Autodesk Fusion 360 part; units mm, degrees
(part 2 of 3)
  line L880 (190.4485, 318.4129) -> (189.5942, 317.9397)
  line L881 (195.3697, 320.9495) -> (194.2984, 320.4242)
  line L882 (211.6798, 327.3307) -> (210.0741, 326.8246)
  line L883 (186.8285, 281.1395) -> (187.261, 279.1724)
  line L884 (184.9285, 291.0204) -> (185.2733, 289.0389)
  line L885 (187.2886, 316.6135) -> (186.3635, 316.0568)
  line L886 (182.4919, 313.4456) -> (182.399, 313.3626)
  line L887 (185.6357, 287.0598) -> (186.0157, 285.0834)
  line L888 (213.3309, 327.826) -> (211.6798, 327.3307)
  line L889 (243.1905, 182.1136) -> (244.2111, 181.3414)
  line L890 (211.4232, 217.808) -> (212.1963, 216.5757)
  line L891 (204.1026, 324.7205) -> (202.7219, 324.1817)
  line L892 (214.5928, 212.9181) -> (215.4171, 211.7129)
  line L893 (186.0157, 285.0834) -> (186.4134, 283.1099)
  line L894 (196.4887, 248.3332) -> (197.2058, 246.4567)
  line L895 (192.2867, 319.3977) -> (191.346, 318.8994)
  line L896 (182.3588, 313.0956) -> (182.3533, 312.8495)
  line L897 (221.5355, 203.5012) -> (222.4584, 202.3634)
  line L898 (228.1911, 331.2302) -> (227.1757, 331.054)
  line L899 (182.734, 313.6258) -> (182.4919, 313.4456)
  line L900 (229.2183, 331.4005) -> (228.1911, 331.2302)
  line L901 (210.0741, 326.8246) -> (208.5136, 326.3091)
  line L902 (198.8469, 322.5569) -> (197.6438, 322.0173)
  line L903 (186.4134, 283.1099) -> (186.8285, 281.1395)
  line L904 (182.3533, 312.8495) -> (182.3576, 312.5288)
  line L905 (205.528, 325.2557) -> (204.1026, 324.7205)
  line L906 (190.7699, 265.5148) -> (191.339, 263.5824)
  line L907 (185.4486, 315.4831) -> (184.5455, 314.8912)
  line L908 (191.346, 318.8994) -> (190.4485, 318.4129)
  line L909 (182.3964, 311.6644) -> (182.4765, 310.5043)
  line L910 (230.2661, 193.6329) -> (231.294, 192.5922)
  line L911 (241.0426, 183.8051) -> (242.1796, 182.8983)
  line L912 (187.261, 279.1724) -> (187.7108, 277.2089)
  line L913 (206.4443, 226.1875) -> (206.7996, 225.5399)
  line L914 (183.2362, 302.9484) -> (183.4731, 300.9569)
  line L915 (194.4344, 254.0045) -> (195.1029, 252.1073)
  line L916 (212.1963, 216.5757) -> (212.9823, 215.3497)
  line L917 (222.4584, 202.3634) -> (223.3933, 201.2354)
  line L918 (184.2925, 294.9899) -> (184.6016, 293.0042)
  line L919 (226.1718, 330.8721) -> (224.199, 330.492)
  line L920 (213.7812, 214.1305) -> (214.5928, 212.9181)
  line L921 (229.2496, 194.6856) -> (230.2661, 193.6329)
  line L922 (231.3075, 331.7228) -> (230.2571, 331.5647)
  line L923 (194.2984, 320.4242) -> (193.2708, 319.9065)
  line L924 (208.9796, 221.8036) -> (209.7164, 220.5848)
  line L925 (200.196, 239.0794) -> (200.5746, 238.1864)
  line L926 (216.254, 210.5152) -> (217.1034, 209.3252)
  line L927 (198.1538, 320.0225) -> (199.198, 320.4971)
  line L928 (237.6951, 186.6124) -> (238.8002, 185.6625)
  line L929 (196.3039, 254.6319) -> (195.6779, 256.4565)
  line L930 (239.9161, 184.7266) -> (241.0426, 183.8051)
  line L931 (186.1932, 295.8614) -> (185.9184, 297.7719)
  line L932 (184.8426, 312.7237) -> (185.3358, 313.0673)
  line L933 (192.5275, 259.7337) -> (193.1466, 257.8179)
  line L934 (191.2359, 271.2561) -> (190.7519, 273.1282)
  line L935 (246.2732, 179.825) -> (248.1998, 178.4241)
  line L936 (191.7358, 269.3885) -> (191.2359, 271.2561)
  line L937 (189.3954, 278.7688) -> (188.9752, 280.6564)
  line L938 (189.8316, 276.8847) -> (189.3954, 278.7688)
  line L939 (189.6821, 269.3948) -> (190.2176, 267.4524)
  line L940 (184.4092, 311.5322) -> (184.3858, 311.947)
  line L941 (198.2755, 249.1965) -> (197.6027, 251.0016)
  line L942 (215.4171, 211.7129) -> (216.254, 210.5152)
  line L943 (195.1029, 252.1073) -> (195.7877, 250.2168)
  line L944 (195.0675, 258.2873) -> (194.4728, 260.124)
  line L945 (244.2111, 181.3414) -> (245.2393, 180.5793)
  line L946 (224.3401, 200.1173) -> (225.2987, 199.0094)
  line L947 (185.1917, 303.5112) -> (184.9822, 305.4263)
  line L948 (188.6623, 273.2934) -> (189.1637, 271.3419)
  line L949 (197.9391, 244.5874) -> (198.6883, 242.7258)
  line L950 (225.2987, 199.0094) -> (226.269, 197.912)
  line L951 (228.2445, 195.7498) -> (229.2496, 194.6856)
  line L952 (207.737, 223.9002) -> (208.3199, 222.9089)
  line L953 (232.3331, 191.5636) -> (233.3834, 190.5474)
  line L954 (195.7877, 250.2168) -> (196.4887, 248.3332)
  line L955 (189.1637, 271.3419) -> (189.6821, 269.3948)
  line L956 (233.3834, 190.5474) -> (234.4449, 189.5439)
  line L957 (218.8395, 206.9696) -> (219.726, 205.8045)
  line L958 (193.7823, 255.9081) -> (194.4344, 254.0045)
  line L959 (217.1034, 209.3252) -> (217.9652, 208.1433)
  line L960 (236.6008, 187.5761) -> (237.6951, 186.6124)
  line L961 (200.9684, 237.3) -> (206.4443, 226.1875)
  line L962 (188.178, 275.2492) -> (188.6623, 273.2934)
  line L963 (196.9455, 252.8135) -> (196.3039, 254.6319)
  line L964 (192.2516, 267.5255) -> (191.7358, 269.3885)
  line L965 (223.3933, 201.2354) -> (224.3401, 200.1173)
  line L966 (191.339, 263.5824) -> (191.9249, 261.6553)
  line L967 (200.5746, 238.1864) -> (200.9684, 237.3)
  line L968 (199.198, 320.4971) -> (200.2826, 320.9764)
  line L969 (188.1829, 284.4416) -> (187.8109, 286.3388)
  line L970 (187.455, 288.2387) -> (187.1153, 290.1411)
  line L971 (193.3307, 263.8142) -> (192.7833, 265.6673)
  line L972 (184.3824, 312.2188) -> (184.3884, 312.3009)
  line L973 (190.2837, 275.0044) -> (189.8316, 276.8847)
  line L974 (192.7833, 265.6673) -> (192.2516, 267.5255)
  line L975 (198.6883, 242.7258) -> (199.4535, 240.8719)
  line L976 (209.7164, 220.5848) -> (210.5308, 219.2528)
  line L977 (206.7996, 225.5399) -> (207.2303, 224.7774)
  line L978 (219.726, 205.8045) -> (220.6247, 204.6483)
  line L979 (210.5308, 219.2528) -> (211.4232, 217.808)
  line L980 (212.9823, 215.3497) -> (213.7812, 214.1305)
  line L981 (208.3199, 222.9089) -> (208.9796, 221.8036)
  line L982 (199.4535, 240.8719) -> (200.196, 239.0794)
  line L983 (207.2303, 224.7774) -> (207.737, 223.9002)
  line L984 (235.5173, 188.5534) -> (236.6008, 187.5761)
  line L985 (231.294, 192.5922) -> (232.3331, 191.5636)
  line L986 (190.2176, 267.4524) -> (190.7699, 265.5148)
  line L987 (191.9249, 261.6553) -> (192.5275, 259.7337)
  line L988 (227.251, 196.8254) -> (228.2445, 195.7498)
  line L989 (238.8002, 185.6625) -> (239.9161, 184.7266)
  line L990 (220.6247, 204.6483) -> (221.5355, 203.5012)
  line L991 (187.8109, 286.3388) -> (187.455, 288.2387)
  line L992 (245.2393, 180.5793) -> (246.2732, 179.825)
  line L993 (294.5657, 322.5161) -> (295.4347, 322.1728)
  line L994 (191.9665, 316.9376) -> (193.5353, 317.764)
  line L995 (278.8099, 327.5376) -> (279.9258, 327.2443)
  line L996 (186.8702, 314.0439) -> (187.9132, 314.6687)
  line L997 (184.4516, 310.9753) -> (184.4092, 311.5322)
  line L998 (238.245, 330.6174) -> (239.0438, 330.7015)
  line L999 (240.3196, 330.8043) -> (258.3534, 330.7921)
  line L1000 (261.8335, 330.4341) -> (263.5877, 330.2118)
  line L1001 (232.6443, 329.8932) -> (235.2057, 330.2411)
  line L1002 (187.1153, 290.1411) -> (186.7917, 292.0458)
  line L1003 (185.9184, 297.7719) -> (185.6598, 299.6838)
  line L1004 (184.3999, 312.3469) -> (184.4429, 312.401)
  line L1005 (187.9132, 314.6687) -> (189.1413, 315.3788)
  line L1006 (184.5888, 309.4382) -> (184.4516, 310.9753)
  line L1007 (197.15, 319.5539) -> (198.1538, 320.0225)
  line L1008 (193.8939, 261.9664) -> (193.3307, 263.8142)
  line L1009 (190.7519, 273.1282) -> (190.2837, 275.0044)
  line L1010 (184.4429, 312.401) -> (184.5309, 312.4822)
  line L1011 (184.3858, 311.947) -> (184.3824, 312.2188)
  line L1012 (248.8662, 177.9546) -> (248.9417, 177.9125)
  line L1013 (210.4325, 324.8283) -> (211.8874, 325.2931)
  line L1014 (206.3175, 323.399) -> (207.6477, 323.88)
  line L1015 (223.2492, 328.2546) -> (225.0422, 328.6208)
  line L1016 (269.5072, 329.3395) -> (270.9528, 329.1031)
  line L1017 (195.6779, 256.4565) -> (195.0675, 258.2873)
  line L1018 (188.9752, 280.6564) -> (188.571, 282.5475)
  line L1019 (195.2628, 318.6395) -> (196.1863, 319.0925)
  line L1020 (258.3534, 330.7921) -> (258.6905, 330.7668)
  line L1021 (270.9528, 329.1031) -> (272.0957, 328.9193)
  line L1022 (218.1261, 327.0605) -> (219.7913, 327.4732)
  line L1023 (194.3791, 318.1963) -> (195.2628, 318.6395)
  line L1024 (239.0438, 330.7015) -> (239.7353, 330.7641)
  line L1025 (275.5164, 328.3239) -> (276.1633, 328.1825)
  line L1026 (259.3837, 330.7039) -> (260.4318, 330.5955)
  line L1027 (283.9678, 326.1106) -> (285.7506, 325.5765)
  line L1028 (198.9639, 247.3984) -> (198.2755, 249.1965)
  line L1029 (295.4347, 322.1728) -> (296.301, 321.8224)
  line L1030 (203.7807, 322.4298) -> (205.0285, 322.9152)
  line L1031 (207.6477, 323.88) -> (209.0193, 324.3568)
  line L1032 (190.5552, 316.1702) -> (191.9665, 316.9376)
  line L1033 (184.9822, 305.4263) -> (184.7891, 307.3421)
  line L1034 (194.4728, 260.124) -> (193.8939, 261.9664)
  line L1035 (185.4176, 301.597) -> (185.1917, 303.5112)
  line L1036 (248.1998, 178.4241) -> (248.7176, 178.0543)
  line L1037 (186.4843, 293.9527) -> (186.1932, 295.8614)
  line L1038 (185.3358, 313.0673) -> (186.0113, 313.5087)
  line L1039 (197.6027, 251.0016) -> (196.9455, 252.8135)
  line L1040 (196.1863, 319.0925) -> (197.15, 319.5539)
  line L1041 (248.7176, 178.0543) -> (248.8662, 177.9546)
  line L1042 (184.3884, 312.3009) -> (184.3999, 312.3469)
  line L1043 (193.5353, 317.764) -> (194.3791, 318.1963)
  line L1044 (184.7891, 307.3421) -> (184.5888, 309.4382)
  line L1045 (188.571, 282.5475) -> (188.1829, 284.4416)
  line L1046 (272.0957, 328.9193) -> (273.2392, 328.7379)
  line L1047 (189.1413, 315.3788) -> (190.5552, 316.1702)
  line L1048 (184.5309, 312.4822) -> (184.8426, 312.7237)
  line L1049 (185.6598, 299.6838) -> (185.4176, 301.597)
  line L1050 (298.8814, 320.7283) -> (299.7349, 320.349)
  line L1051 (300.5849, 319.9624) -> (301.4312, 319.5683)
  line L1052 (211.8874, 325.2931) -> (213.384, 325.7499)
  line L1053 (186.0113, 313.5087) -> (186.8702, 314.0439)
  line L1054 (186.7917, 292.0458) -> (186.4843, 293.9527)
  line L1055 (209.0193, 324.3568) -> (210.4325, 324.8283)
  line L1056 (265.6932, 329.921) -> (268.1486, 329.554)
  line L1057 (277.8105, 327.7908) -> (278.8099, 327.5376)
  line L1058 (239.7353, 330.7641) -> (240.3196, 330.8043)
  line L1059 (202.5738, 321.944) -> (203.7807, 322.4298)
  line L1060 (260.4318, 330.5955) -> (261.8335, 330.4341)
  line L1061 (228.757, 329.298) -> (230.679, 329.6065)
  line L1062 (291.064, 323.8204) -> (292.8196, 323.182)
  line L1063 (298.0244, 321.1002) -> (298.8814, 320.7283)
  line L1064 (313.6797, 306.995) -> (313.501, 305.1643)
  line L1065 (302.2738, 319.1668) -> (303.1123, 318.7576)
  line L1066 (313.8935, 309.2436) -> (313.6797, 306.995)
  line L1067 (312.0915, 294.2029) -> (311.8012, 292.3814)
  line L1068 (273.2392, 328.7379) -> (274.3804, 328.5443)
  line L1069 (276.9282, 328.0053) -> (277.8105, 327.7908)
  line L1070 (219.7913, 327.4732) -> (221.499, 327.8716)
  line L1071 (305.6295, 265.399) -> (305.1009, 263.6307)
  line L1072 (312.4719, 313.4707) -> (313.3652, 312.9061)
  line L1073 (314.1337, 311.9322) -> (314.0498, 310.8908)
  line L1074 (313.306, 303.3344) -> (313.095, 301.5055)
  line L1075 (299.7349, 320.349) -> (300.5849, 319.9624)
  line L1076 (313.9209, 312.5379) -> (314.0694, 312.4265)
  line L1077 (201.4079, 321.4591) -> (202.5738, 321.944)
  line L1078 (301.0102, 251.3972) -> (300.3711, 249.6723)
  line L1079 (307.2409, 316.5958) -> (308.0528, 316.1398)
  line L1080 (221.499, 327.8716) -> (223.2492, 328.2546)
  line L1081 (226.8781, 328.9691) -> (228.757, 329.298)
  line L1082 (292.8196, 323.182) -> (294.5657, 322.5161)
  line L1083 (258.6905, 330.7668) -> (259.3837, 330.7039)
  line L1084 (214.9226, 326.1977) -> (216.5032, 326.6349)
  line L1085 (205.0285, 322.9152) -> (206.3175, 323.399)
  line L1086 (230.679, 329.6065) -> (232.6443, 329.8932)
  line L1087 (263.5877, 330.2118) -> (265.6932, 329.921)
  line L1088 (268.1486, 329.554) -> (269.5072, 329.3395)
  line L1089 (274.3804, 328.5443) -> (274.9492, 328.4384)
  line L1090 (308.9263, 277.8968) -> (308.4991, 276.0998)
  line L1091 (305.6029, 317.484) -> (306.4242, 317.0439)
  line L1092 (307.1295, 270.7309) -> (306.6439, 268.9492)
  line L1093 (312.6249, 297.8512) -> (312.3661, 296.0262)
  line L1094 (309.6616, 315.2036) -> (310.4583, 314.7233)
  line L1095 (311.4954, 290.5619) -> (311.1741, 288.7447)
  line L1096 (310.4854, 285.1174) -> (310.1182, 283.3078)
  line L1097 (310.1182, 283.3078) -> (309.7359, 281.501)
  line L1098 (305.1009, 263.6307) -> (304.5582, 261.8672)
  line L1099 (303.9468, 318.3408) -> (304.777, 317.9163)
  line L1100 (213.384, 325.7499) -> (214.9226, 326.1977)
  line L1101 (279.9258, 327.2443) -> (281.1578, 326.9097)
  line L1102 (308.0528, 316.1398) -> (308.8598, 315.6758)
  line L1103 (287.5283, 325.0171) -> (289.2998, 324.4319)
  line L1104 (311.8012, 292.3814) -> (311.4954, 290.5619)
  line L1105 (282.5052, 326.5322) -> (283.9678, 326.1106)
  line L1106 (314.1303, 312.3631) -> (314.1401, 312.3128)
  line L1107 (274.9492, 328.4384) -> (275.5164, 328.3239)
  line L1108 (200.2826, 320.9764) -> (201.4079, 321.4591)
  line L1109 (237.339, 330.5122) -> (238.245, 330.6174)
  line L1110 (216.5032, 326.6349) -> (218.1261, 327.0605)
  line L1111 (281.1578, 326.9097) -> (282.5052, 326.5322)
  line L1112 (285.7506, 325.5765) -> (287.5283, 325.0171)
  line L1113 (276.1633, 328.1825) -> (276.9282, 328.0053)
  line L1114 (289.2998, 324.4319) -> (291.064, 323.8204)
  line L1115 (297.1643, 321.4649) -> (298.0244, 321.1002)
  line L1116 (225.0422, 328.6208) -> (226.8781, 328.9691)
  line L1117 (235.2057, 330.2411) -> (237.339, 330.5122)
  line L1118 (296.301, 321.8224) -> (297.1643, 321.4649)
  line L1119 (306.6439, 268.9492) -> (306.1438, 267.1719)
  line L1120 (314.1401, 312.3128) -> (314.1439, 312.2242)
  line L1121 (236.8455, 190.0948) -> (235.7247, 191.1305)
  line L1122 (310.4583, 314.7233) -> (311.2496, 314.2347)
  line L1123 (308.4991, 276.0998) -> (308.0572, 274.3063)
  line L1124 (306.1438, 267.1719) -> (305.6295, 265.399)
  line L1125 (303.4307, 258.3554) -> (302.8462, 256.6074)
  line L1126 (279.9298, 210.7253) -> (278.7353, 209.0622)
  line L1127 (249.2499, 180.1523) -> (249.1978, 180.174)
  line L1128 (256.2407, 185.4395) -> (255.1379, 184.5517)
  line L1129 (313.095, 301.5055) -> (312.8679, 299.6777)
  line L1130 (296.9792, 241.1186) -> (296.282, 239.4885)
  line L1131 (288.4746, 223.9458) -> (287.906, 222.9657)
  line L1132 (313.3652, 312.9061) -> (313.9209, 312.5379)
  line L1133 (302.8462, 256.6074) -> (302.2478, 254.8649)
  line L1134 (303.1123, 318.7576) -> (303.9468, 318.3408)
  line L1135 (302.2478, 254.8649) -> (301.6358, 253.1281)
  line L1136 (295.0943, 236.8299) -> (294.6113, 235.7987)
  line L1137 (261.7197, 190.1093) -> (259.4933, 188.169)
  line L1138 (314.1109, 312.3888) -> (314.1303, 312.3631)
  line L1139 (249.3666, 180.2174) -> (249.2896, 180.1687)
  line L1140 (237.9781, 189.0732) -> (236.8455, 190.0948)
  line L1141 (265.5721, 193.6166) -> (264.9971, 193.0698)
  line L1142 (264.9971, 193.0698) -> (264.3244, 192.4454)
  line L1143 (234.6159, 192.1801) -> (233.5192, 193.2433)
  line L1144 (281.1036, 212.4027) -> (279.9298, 210.7253)
  line L1145 (288.9441, 224.778) -> (288.4746, 223.9458)
  line L1146 (309.7359, 281.501) -> (309.3385, 279.6973)
  line L1147 (301.6358, 253.1281) -> (301.0102, 251.3972)
  line L1148 (308.8598, 315.6758) -> (309.6616, 315.2036)
  line L1149 (250.627, 181.1318) -> (249.6337, 180.4076)
  line L1150 (257.334, 186.3388) -> (256.2407, 185.4395)
  line L1151 (233.5192, 193.2433) -> (232.4347, 194.3197)
  line L1152 (232.4347, 194.3197) -> (231.3627, 195.4091)
  line L1153 (313.501, 305.1643) -> (313.306, 303.3344)
  line L1154 (278.1296, 208.2367) -> (277.5179, 207.4156)
  line L1155 (307.6006, 272.5166) -> (307.1295, 270.7309)
  line L1156 (242.6238, 185.134) -> (241.4454, 186.0962)
  line L1157 (254.0255, 183.6763) -> (252.903, 182.814)
  line L1158 (245.0138, 183.2568) -> (243.8133, 184.1875)
  line L1159 (272.3827, 201.043) -> (266.0497, 194.0855)
  line L1160 (314.0498, 310.8908) -> (313.8935, 309.2436)
  line L1161 (301.4312, 319.5683) -> (302.2738, 319.1668)
  line L1162 (249.0969, 180.2383) -> (248.7472, 180.4891)
  line L1163 (314.1439, 312.2242) -> (314.1337, 311.9322)
  line L1164 (298.562, 244.9862) -> (297.7405, 242.9507)
  line L1165 (297.7405, 242.9507) -> (296.9792, 241.1186)
  line L1166 (239.1223, 188.066) -> (237.9781, 189.0732)
  line L1167 (314.0694, 312.4265) -> (314.1109, 312.3888)
  line L1168 (308.0572, 274.3063) -> (307.6006, 272.5166)
  line L1169 (311.1741, 288.7447) -> (310.8374, 286.9298)
  line L1170 (299.4401, 247.2263) -> (298.562, 244.9862)
  line L1171 (312.3661, 296.0262) -> (312.0915, 294.2029)
  line L1172 (310.8374, 286.9298) -> (310.4854, 285.1174)
  line L1173 (309.3385, 279.6973) -> (308.9263, 277.8968)
  line L1174 (304.5582, 261.8672) -> (304.0014, 260.1087)
  line L1175 (306.4242, 317.0439) -> (307.2409, 316.5958)
  line L1176 (312.8679, 299.6777) -> (312.6249, 297.8512)
  line L1177 (311.2496, 314.2347) -> (312.4719, 313.4707)
  line L1178 (300.3711, 249.6723) -> (299.4401, 247.2263)
  line L1179 (304.777, 317.9163) -> (305.6029, 317.484)
  line L1180 (295.6525, 238.0594) -> (295.0943, 236.8299)
  line L1181 (304.0014, 260.1087) -> (303.4307, 258.3554)
  line L1182 (296.282, 239.4885) -> (295.6525, 238.0594)
  line L1183 (274.3625, 203.3875) -> (273.7102, 202.5994)
  line L1184 (249.2896, 180.1687) -> (249.2499, 180.1523)
  line L1185 (287.2355, 221.8397) -> (286.4604, 220.5699)
  line L1186 (243.8133, 184.1875) -> (242.6238, 185.134)
  line L1187 (248.7472, 180.4891) -> (247.4471, 181.4443)
  line L1188 (273.7102, 202.5994) -> (273.0504, 201.8178)
  line L1189 (251.7703, 181.9656) -> (250.627, 181.1318)
  line L1190 (247.4471, 181.4443) -> (246.2251, 182.3423)
  line L1191 (283.4796, 215.9172) -> (282.2584, 214.0919)
  line L1192 (264.3244, 192.4454) -> (263.5541, 191.7437)
  line L1193 (273.0504, 201.8178) -> (272.3827, 201.043)
  line L1194 (230.3032, 196.5112) -> (229.2564, 197.6257)
  line L1195 (196.1486, 220.6446) -> (196.7783, 219.3402)
  line L1196 (187.8279, 240.6292) -> (188.3178, 239.2788)
  line L1197 (222.2966, 205.7499) -> (221.3566, 206.9532)
  line L1198 (221.3566, 206.9532) -> (220.4307, 208.1662)
  line L1199 (228.2225, 198.7523) -> (227.2015, 199.8907)
  line L1200 (258.4181, 187.2489) -> (257.334, 186.3388)
  line L1201 (284.5852, 217.6066) -> (283.4796, 215.9172)
  line L1202 (287.906, 222.9657) -> (287.2355, 221.8397)
  line L1203 (282.2584, 214.0919) -> (281.1036, 212.4027)
  line L1204 (199.3927, 214.1694) -> (200.0703, 212.8894)
  line L1205 (218.6213, 210.6205) -> (217.7382, 211.8612)
  line L1206 (276.9001, 206.5994) -> (276.2759, 205.7881)
  line L1207 (255.1379, 184.5517) -> (254.0255, 183.6763)
  line L1208 (202.1609, 209.0826) -> (202.8772, 207.8253)
  line L1209 (276.2759, 205.7881) -> (275.6451, 204.9822)
  line L1210 (190.3692, 233.8971) -> (190.9051, 232.5575)
  line L1211 (275.6451, 204.9822) -> (275.0073, 204.1819)
  line L1212 (208.2063, 227.1364) -> (202.7875, 238.1331)
  line L1213 (277.5179, 207.4156) -> (276.9001, 206.5994)
  line L1214 (286.4604, 220.5699) -> (285.5778, 219.1582)
  line L1215 (249.6337, 180.4076) -> (249.3666, 180.2174)
  line L1216 (215.177, 215.6338) -> (214.3531, 216.9072)
  line L1217 (259.4933, 188.169) -> (258.4181, 187.2489)
  line L1218 (249.1978, 180.174) -> (249.0969, 180.2383)
  line L1219 (210.648, 222.9706) -> (210.0287, 224.007)
  line L1220 (198.0664, 216.745) -> (198.7247, 215.4547)
  line L1221 (219.5188, 209.3888) -> (218.6213, 210.6205)
  line L1222 (231.3627, 195.4091) -> (230.3032, 196.5112)
  line L1223 (229.2564, 197.6257) -> (228.2225, 198.7523)
  line L1224 (235.7247, 191.1305) -> (234.6159, 192.1801)
  line L1225 (275.0073, 204.1819) -> (274.3625, 203.3875)
  line L1226 (241.4454, 186.0962) -> (240.2782, 187.0736)
  line L1227 (294.6113, 235.7987) -> (288.9441, 224.778)
  line L1228 (285.5778, 219.1582) -> (284.5852, 217.6066)
  line L1229 (246.2251, 182.3423) -> (245.0138, 183.2568)
  line L1230 (262.6859, 190.9648) -> (261.7197, 190.1093)
  line L1231 (252.903, 182.814) -> (251.7703, 181.9656)
  line L1232 (278.7353, 209.0622) -> (278.1296, 208.2367)
  line L1233 (266.0497, 194.0855) -> (265.5721, 193.6166)
  line L1234 (263.5541, 191.7437) -> (262.6859, 190.9648)
  line L1235 (240.2782, 187.0736) -> (239.1223, 188.066)
  line L1236 (174.1164, 303.7009) -> (174.2775, 301.8868)
  line L1237 (186.2399, 321.8008) -> (184.9873, 321.0676)
  line L1238 (178.5913, 316.5626) -> (178.4678, 316.4358)
  line L1239 (187.5035, 322.517) -> (186.2399, 321.8008)
  line L1240 (193.975, 325.8444) -> (192.6615, 325.2125)
  line L1241 (192.6615, 325.2125) -> (191.3572, 324.5639)
  line L1242 (182.6702, 319.6432) -> (181.7405, 319.0373)
  line L1243 (178.8282, 316.8304) -> (178.5913, 316.5626)
  line L1244 (173.6704, 311.437) -> (173.6724, 310.891)
  line L1245 (204.7741, 330.3046) -> (203.3992, 329.8043)
  line L1246 (178.4678, 316.4358) -> (178.3376, 316.3185)
  line L1247 (175.0547, 314.1173) -> (174.9008, 313.9498)
  line L1248 (179.0683, 317.0917) -> (178.8282, 316.8304)
  line L1249 (184.9873, 321.0676) -> (183.7461, 320.3171)
  line L1250 (175.7475, 314.7115) -> (175.565, 314.5732)
  line L1251 (173.7655, 308.4261) -> (173.8352, 307.3306)
  line L1252 (180.9539, 318.5041) -> (180.3076, 318.0482)
  line L1253 (173.969, 305.5156) -> (174.1164, 303.7009)
  line L1254 (179.4245, 317.3873) -> (179.0683, 317.0917)
  line L1255 (173.687, 310.2069) -> (173.7171, 309.3851)
  line L1256 (173.7171, 309.3851) -> (173.7655, 308.4261)
  line L1257 (196.6284, 327.0581) -> (195.2974, 326.4595)
  line L1258 (177.6023, 315.892) -> (177.1697, 315.6333)
  line L1259 (174.9008, 313.9498) -> (173.7111, 312.2406)
  line L1260 (176.3173, 315.0933) -> (175.9345, 314.8439)
  line L1261 (173.6926, 312.1123) -> (173.6781, 311.8442)
  line L1262 (173.6781, 311.8442) -> (173.6704, 311.437)
  line L1263 (179.7988, 317.6744) -> (179.4245, 317.3873)
  line L1264 (208.9336, 331.7091) -> (207.5416, 331.257)
  line L1265 (176.7433, 315.3633) -> (176.3173, 315.0933)
  line L1266 (266.3752, 170.6581) -> (267.2926, 171.498)
  line L1267 (274.9089, 179.1627) -> (276.0833, 180.4296)
  line L1268 (295.5565, 206.839) -> (296.4858, 208.4271)
  line L1269 (247.5941, 159.0159) -> (248.0084, 158.937)
  line L1270 (183.5972, 253.6008) -> (184.119, 251.8565)
  line L1271 (178.1982, 316.2147) -> (178.0471, 316.128)
  line L1272 (176.9367, 282.0055) -> (177.2577, 280.2083)
  line L1273 (183.0875, 255.3495) -> (183.5972, 253.6008)
  line L1274 (181.6318, 260.6201) -> (182.1047, 258.8593)
  line L1275 (174.4523, 300.0734) -> (174.6406, 298.2608)
  line L1276 (177.9384, 276.621) -> (178.2981, 274.831)
  line L1277 (271.7648, 175.8739) -> (272.7484, 176.886)
  line L1278 (176.6288, 283.8048) -> (176.9367, 282.0055)
  line L1279 (183.7461, 320.3171) -> (182.6702, 319.6432)
  line L1280 (182.59, 257.1024) -> (183.0875, 255.3495)
  line L1281 (175.5284, 291.021) -> (175.7837, 289.2144)
  line L1282 (188.7779, 323.2162) -> (187.5035, 322.517)
  line L1283 (180.2874, 265.9246) -> (180.7231, 264.1529)
  line L1284 (249.1223, 158.8451) -> (249.4296, 158.8614)
  line L1285 (176.334, 285.6062) -> (176.6288, 283.8048)
  line L1286 (269.2152, 173.3293) -> (269.997, 174.0968)
  line L1287 (181.1712, 262.3847) -> (181.6318, 260.6201)
  line L1288 (182.1047, 258.8593) -> (182.59, 257.1024)
  line L1289 (179.8643, 267.6997) -> (180.2874, 265.9246)
  line L1290 (263.386, 168.1122) -> (264.4041, 168.961)
  line L1291 (270.8473, 174.9446) -> (271.7648, 175.8739)
  line L1292 (252.9334, 160.1604) -> (253.1909, 160.33)
  line L1293 (173.8352, 307.3306) -> (173.969, 305.5156)
  line L1294 (174.8424, 296.4491) -> (175.0577, 294.6384)
  line L1295 (286.4775, 193.0809) -> (287.5505, 194.5587)
  line L1296 (175.7837, 289.2144) -> (176.0522, 287.4094)
  line L1297 (174.2775, 301.8868) -> (174.4523, 300.0734)
  line L1298 (177.2577, 280.2083) -> (177.5916, 278.4134)
  line L1299 (176.0522, 287.4094) -> (176.334, 285.6062)
  line L1300 (178.6706, 273.0438) -> (179.0558, 271.2594)
  line L1301 (179.0558, 271.2594) -> (179.4537, 269.478)
  line L1302 (178.2981, 274.831) -> (178.6706, 273.0438)
  line L1303 (264.4041, 168.961) -> (265.4584, 169.8515)
  line L1304 (180.7231, 264.1529) -> (181.1712, 262.3847)
  line L1305 (262.4046, 167.3047) -> (263.386, 168.1122)
  line L1306 (277.3044, 181.7743) -> (278.5088, 183.1349)
  line L1307 (268.5031, 172.6412) -> (269.2152, 173.3293)
  line L1308 (195.2974, 326.4595) -> (193.975, 325.8444)
  line L1309 (180.3076, 318.0482) -> (179.7988, 317.6744)
  line L1310 (184.119, 251.8565) -> (184.653, 250.1165)
  line L1311 (278.5088, 183.1349) -> (279.6965, 184.5111)
  line L1312 (248.8155, 158.8477) -> (249.1223, 158.8451)
  line L1313 (261.4602, 166.5378) -> (262.4046, 167.3047)
  line L1314 (175.0577, 294.6384) -> (175.2864, 292.829)
  line L1315 (179.4537, 269.478) -> (179.8643, 267.6997)
  line L1316 (269.997, 174.0968) -> (270.8473, 174.9446)
  line L1317 (249.7369, 158.8955) -> (250.0435, 158.9465)
  line L1318 (284.2827, 190.1666) -> (285.3882, 191.6168)
  line L1319 (174.6406, 298.2608) -> (174.8424, 296.4491)
  line L1320 (175.2864, 292.829) -> (175.5284, 291.021)
  line L1321 (258.0633, 163.8677) -> (259.6848, 165.1243)
  line L1322 (177.5916, 278.4134) -> (177.9384, 276.621)
  line L1323 (283.1608, 188.7307) -> (284.2827, 190.1666)
  line L1324 (253.1909, 160.33) -> (254.1596, 160.9991)
  line L1325 (282.0225, 187.3093) -> (283.1608, 188.7307)
  line L1326 (291.6813, 200.6008) -> (292.674, 202.1427)
  line L1327 (252.3962, 159.8393) -> (252.6683, 159.9964)
  line L1328 (292.674, 202.1427) -> (293.6507, 203.6966)
  line L1329 (207.5416, 331.257) -> (206.155, 330.7888)
  line L1330 (256.5994, 162.764) -> (258.0633, 163.8677)
  line L1331 (288.6074, 196.0499) -> (289.6481, 197.5541)
  line L1332 (318.6482, 265.2318) -> (319.0725, 267.0306)
  line L1333 (280.8678, 185.9026) -> (282.0225, 187.3093)
  line L1334 (273.7968, 177.9818) -> (274.9089, 179.1627)
  line L1335 (319.8793, 270.6315) -> (320.262, 272.4332)
  line L1336 (251.5442, 159.4185) -> (251.8335, 159.5493)
  line L1337 (251.8335, 159.5493) -> (252.1177, 159.6899)
  line L1338 (290.6727, 199.0712) -> (291.6813, 200.6008)
  line L1339 (299.1794, 213.2553) -> (300.0461, 214.8851)
  line L1340 (316.3158, 256.267) -> (316.8106, 258.0552)
  line L1341 (301.7331, 218.1735) -> (302.5534, 219.8316)
  line L1342 (317.7576, 261.6393) -> (318.2099, 263.4347)
  line L1343 (300.8973, 216.5246) -> (301.7331, 218.1735)
  line L1344 (297.3993, 210.0261) -> (298.2972, 211.6355)
  line L1345 (298.2972, 211.6355) -> (299.1794, 213.2553)
  line L1346 (259.6848, 165.1243) -> (260.5535, 165.8112)
  line L1347 (317.2912, 259.8461) -> (317.7576, 261.6393)
  line L1348 (267.2926, 171.498) -> (268.5031, 172.6412)
  line L1349 (307.869, 231.6709) -> (308.5681, 233.392)
  line L1350 (254.1596, 160.9991) -> (255.297, 161.8091)
  line L1351 (309.9214, 236.854) -> (310.5758, 238.5942)
  line L1352 (304.9226, 224.858) -> (305.6819, 226.5498)
  line L1353 (300.0461, 214.8851) -> (300.8973, 216.5246)
  line L1354 (323.4129, 291.0258) -> (323.6758, 293.1237)
  line L1355 (308.5681, 233.392) -> (309.2522, 235.1198)
  line L1356 (315.2835, 252.6998) -> (315.8068, 254.4818)
  line L1357 (252.6683, 159.9964) -> (252.9334, 160.1604)
  line L1358 (320.262, 272.4332) -> (320.6309, 274.2353)
  line L1359 (324.1558, 297.3252) -> (324.3764, 299.4281)
  line L1360 (314.7458, 250.9213) -> (315.2835, 252.6998)
  line L1361 (255.297, 161.8091) -> (256.5994, 162.764)
  line L1362 (248.51, 158.8701) -> (248.8155, 158.8477)
  line L1363 (310.5758, 238.5942) -> (311.2154, 240.3401)
  line L1364 (320.6309, 274.2353) -> (320.986, 276.0375)
  line L1365 (250.6521, 159.0949) -> (250.9529, 159.1903)
  line L1366 (311.8403, 242.0916) -> (312.4505, 243.8482)
  line L1367 (249.4296, 158.8614) -> (249.7369, 158.8955)
  line L1368 (293.6507, 203.6966) -> (294.6115, 205.2621)
  line L1369 (247.0305, 159.1815) -> (247.2679, 159.0998)
  line L1370 (260.5535, 165.8112) -> (261.4602, 166.5378)
  line L1371 (303.3584, 221.4986) -> (304.1481, 223.1741)
  line L1372 (252.1177, 159.6899) -> (252.3962, 159.8393)
  line L1373 (296.4858, 208.4271) -> (297.3993, 210.0261)
  line L1374 (265.7606, 170.1123) -> (266.3752, 170.6581)
  line L1375 (279.6965, 184.5111) -> (280.8678, 185.9026)
  line L1376 (272.7484, 176.886) -> (273.7968, 177.9818)
  line L1377 (251.2505, 159.2985) -> (251.5442, 159.4185)
  line L1378 (324.3764, 299.4281) -> (324.5868, 301.5321)
  line L1379 (250.0435, 158.9465) -> (250.3488, 159.0133)
  line L1380 (250.9529, 159.1903) -> (251.2505, 159.2985)
  line L1381 (276.0833, 180.4296) -> (277.3044, 181.7743)
  line L1382 (285.3882, 191.6168) -> (286.4775, 193.0809)
  line L1383 (265.4584, 169.8515) -> (265.7606, 170.1123)
  line L1384 (248.0084, 158.937) -> (248.51, 158.8701)
  line L1385 (306.426, 228.2495) -> (307.155, 229.9566)
  line L1386 (313.0462, 245.6098) -> (313.6272, 247.376)
  line L1387 (294.6115, 205.2621) -> (295.5565, 206.839)
  line L1388 (287.5505, 194.5587) -> (288.6074, 196.0499)
  line L1389 (289.6481, 197.5541) -> (290.6727, 199.0712)
  line L1390 (250.3488, 159.0133) -> (250.6521, 159.0949)
  line L1391 (247.2679, 159.0998) -> (247.5941, 159.0159)
  line L1392 (313.6272, 247.376) -> (314.1937, 249.1466)
  line L1393 (320.986, 276.0375) -> (321.3275, 277.8396)
  line L1394 (319.4829, 268.8306) -> (319.8793, 270.6315)
  line L1395 (311.2154, 240.3401) -> (311.8403, 242.0916)
  line L1396 (312.4505, 243.8482) -> (313.0462, 245.6098)
  line L1397 (302.5534, 219.8316) -> (303.3584, 221.4986)
  line L1398 (315.8068, 254.4818) -> (316.3158, 256.267)
  line L1399 (319.0725, 267.0306) -> (319.4829, 268.8306)
  line L1400 (321.6553, 279.6412) -> (321.9696, 281.4422)
  line L1401 (322.2703, 283.2421) -> (322.5576, 285.0408)
  line L1402 (318.2099, 263.4347) -> (318.6482, 265.2318)
  line L1403 (321.3275, 277.8396) -> (321.6553, 279.6412)
  line L1404 (316.8106, 258.0552) -> (317.2912, 259.8461)
  line L1405 (322.5576, 285.0408) -> (322.8315, 286.8379)
  line L1406 (321.9696, 281.4422) -> (322.2703, 283.2421)
  line L1407 (309.2522, 235.1198) -> (309.9214, 236.854)
  line L1408 (323.9229, 295.2236) -> (324.1558, 297.3252)
  line L1409 (232.6196, 294.0264) -> (232.7551, 294.2154)
  line L1410 (207.0531, 304.9045) -> (207.2431, 305.066)
  line L1411 (205.7789, 304.1295) -> (205.9207, 304.1857)
  line L1412 (322.8315, 286.8379) -> (323.132, 288.9305)
  line L1413 (207.4407, 305.2465) -> (207.6451, 305.4471)
  line L1414 (304.1481, 223.1741) -> (304.9226, 224.858)
  line L1415 (323.132, 288.9305) -> (323.4129, 291.0258)
  line L1416 (314.1937, 249.1466) -> (314.7458, 250.9213)
  line L1417 (305.6819, 226.5498) -> (306.426, 228.2495)
  line L1418 (323.6758, 293.1237) -> (323.9229, 295.2236)
  line L1419 (307.155, 229.9566) -> (307.869, 231.6709)
  line L1420 (218.5146, 292.203) -> (230.3584, 292.201)
  line L1421 (232.2269, 293.5705) -> (232.4447, 293.8101)
  line L1422 (230.3584, 292.201) -> (230.5081, 292.2638)
  line L1423 (216.6625, 295.33) -> (215.7438, 294.9748)
  line L1424 (232.7551, 294.2154) -> (232.8548, 294.3736)
  line L1425 (206.6999, 304.6352) -> (206.8718, 304.7613)
  line L1426 (216.79, 293.2545) -> (218.5146, 292.203)
  line L1427 (208.3709, 306.4019) -> (208.433, 306.5325)
  line L1428 (208.1065, 305.9744) -> (208.2086, 306.1219)
  line L1429 (232.9746, 294.625) -> (232.6923, 295.3607)
  line L1430 (207.8553, 305.6688) -> (207.9891, 305.8231)
  line L1431 (206.3885, 304.4308) -> (206.6999, 304.6352)
  line L1432 (197.7448, 292.201) -> (200.6552, 292.201)
  line L1433 (232.8548, 294.3736) -> (232.9222, 294.497)
  line L1434 (208.2964, 306.2647) -> (208.3709, 306.4019)
  line L1435 (206.8718, 304.7613) -> (207.0531, 304.9045)
  line L1436 (208.2086, 306.1219) -> (208.2964, 306.2647)
  line L1437 (207.9891, 305.8231) -> (208.1065, 305.9744)
  line L1438 (215.7438, 294.9748) -> (216.79, 293.2545)
  line L1439 (231.3388, 292.7855) -> (231.6363, 293.0228)
  line L1440 (232.6923, 295.3607) -> (216.6625, 295.33)
  line L1441 (207.6451, 305.4471) -> (207.8553, 305.6688)
  line L1442 (208.433, 306.5325) -> (208.5242, 306.7707)
  line L1443 (230.6547, 292.3384) -> (230.8444, 292.4475)
  line L1444 (231.9627, 293.3111) -> (232.2269, 293.5705)
  line L1445 (208.5242, 306.7707) -> (208.5778, 306.9719)
  line L1446 (200.6552, 292.201) -> (200.6552, 304.1073)
  line L1447 (200.6552, 304.1073) -> (205.7086, 304.1073)
  line L1448 (205.9207, 304.1857) -> (206.1263, 304.2835)
  line L1449 (230.5081, 292.2638) -> (230.6547, 292.3384)
  line L1450 (207.2431, 305.066) -> (207.4407, 305.2465)
  line L1451 (206.1263, 304.2835) -> (206.3885, 304.4308)
  line L1452 (189.785, 307.0047) -> (189.8056, 306.8714)
  line L1453 (241.3875, 292.201) -> (257.8052, 292.201)
  line L1454 (192.5909, 304.1373) -> (192.6914, 304.1073)
  line L1455 (191.9423, 304.4947) -> (192.1242, 304.3851)
  line L1456 (257.8052, 301.1878) -> (244.4437, 301.3292)
  line L1457 (244.1631, 295.0855) -> (243.8891, 294.934)
  line L1458 (254.2333, 295.3435) -> (244.8724, 295.4061)
  line L1459 (306.7531, 292.201) -> (306.7531, 301.1403)
  line L1460 (306.7531, 301.1403) -> (305.8807, 301.475)
  line L1461 (208.6041, 307.235) -> (208.5927, 307.2823)
  line L1462 (208.5927, 307.2823) -> (189.8073, 307.2823)
  line L1463 (189.8475, 306.7185) -> (189.9162, 306.5489)
  line L1464 (191.6555, 304.6705) -> (191.9423, 304.4947)
  line L1465 (208.6018, 307.1291) -> (208.6041, 307.235)
  line L1466 (190.4092, 305.8156) -> (190.6301, 305.5568)
  line L1467 (190.2046, 306.0858) -> (190.4092, 305.8156)
  line L1468 (244.8724, 295.4061) -> (244.728, 295.3539)
  line L1469 (303.8427, 292.201) -> (306.7531, 292.201)
  line L1470 (189.7862, 307.2006) -> (189.7804, 307.1155)
  line L1471 (243.2234, 294.5213) -> (243.003, 294.3643)
  line L1472 (189.9162, 306.5489) -> (190.0171, 306.3656)
  line L1473 (189.7969, 307.2572) -> (189.7862, 307.2006)
  line L1474 (232.4447, 293.8101) -> (232.6196, 294.0264)
  line L1475 (191.3799, 304.8663) -> (191.6555, 304.6705)
  line L1476 (231.6363, 293.0228) -> (231.9627, 293.3111)
  line L1477 (230.8444, 292.4475) -> (231.0736, 292.5951)
  line L1478 (208.5778, 306.9719) -> (208.6018, 307.1291)
  line L1479 (241.401, 298.2865) -> (254.8948, 298.2865)
  line L1480 (231.0736, 292.5951) -> (231.3388, 292.7855)
  line L1481 (232.9222, 294.497) -> (232.9746, 294.625)
  line L1482 (244.728, 295.3539) -> (244.3954, 295.2041)
  line L1483 (189.8073, 307.2823) -> (189.7969, 307.2572)
  line L1484 (244.4438, 301.3292) -> (244.2838, 304.1073)
  line L1485 (192.1242, 304.3851) -> (192.3062, 304.274)
  line L1486 (257.788, 306.8648) -> (257.1438, 307.2742)
  line L1487 (290.349, 292.201) -> (293.2594, 292.201)
  line L1488 (192.4936, 304.1764) -> (192.5909, 304.1373)
  line L1489 (293.2594, 298.2865) -> (303.8427, 298.2865)
  line L1490 (189.7804, 307.1155) -> (189.785, 307.0047)
  line L1491 (254.8948, 298.2865) -> (254.8948, 295.376)
  line L1492 (191.1164, 305.0805) -> (191.3799, 304.8663)
  line L1493 (256.7676, 305.187) -> (257.788, 306.8648)
  line L1494 (192.6914, 304.1073) -> (197.7448, 304.1073)
  line L1495 (257.8052, 292.201) -> (257.8052, 301.1878)
  line L1496 (305.8807, 301.475) -> (290.349, 301.4319)
  line L1497 (303.8427, 298.2865) -> (303.8427, 292.201)
  line L1498 (189.8056, 306.8714) -> (189.8475, 306.7185)
  line L1499 (244.2838, 304.1073) -> (254.6513, 304.1073)
  line L1500 (190.6301, 305.5568) -> (190.8662, 305.3112)
  line L1501 (190.8662, 305.3112) -> (191.1164, 305.0805)
  line L1502 (254.8011, 295.3348) -> (254.6527, 295.3294)
  line L1503 (243.5753, 294.7469) -> (243.2234, 294.5213)
  line L1504 (244.3954, 295.2041) -> (244.1631, 295.0855)
  line L1505 (205.7086, 304.1073) -> (205.7789, 304.1295)
  line L1506 (257.1438, 307.2742) -> (241.401, 307.2823)
  line L1507 (197.7448, 304.1073) -> (197.7448, 292.201)
  line L1508 (241.401, 307.2823) -> (241.401, 298.2865)
  line L1509 (254.6513, 304.1073) -> (256.7676, 305.187)
  line L1510 (293.2594, 292.201) -> (293.2594, 298.2865)
  line L1511 (254.4599, 295.3391) -> (254.2333, 295.3435)
  line L1512 (254.8948, 295.376) -> (254.8555, 295.3497)
  line L1513 (243.8891, 294.934) -> (243.5753, 294.7469)
  line L1514 (192.3062, 304.274) -> (192.4936, 304.1764)
  line L1515 (243.003, 294.3643) -> (242.7924, 294.1926)
  line L1516 (232.2269, 299.6559) -> (232.4447, 299.8956)
  line L1517 (279.2627, 292.201) -> (280.8474, 293.0205)
  line L1518 (304.1421, 304.1073) -> (304.3182, 304.1655)
  line L1519 (281.8823, 295.4139) -> (281.8537, 295.4187)
  line L1520 (281.8985, 295.3434) -> (281.8823, 295.4139)
  line L1521 (230.5081, 298.3492) -> (230.6547, 298.4238)
  line L1522 (281.5595, 295.3866) -> (281.1925, 295.3484)
  line L1523 (241.9043, 293.161) -> (241.764, 292.9293)
  line L1524 (281.1925, 295.3484) -> (280.6917, 295.3175)
  line L1525 (304.7393, 304.3895) -> (304.9827, 304.5526)
  line L1526 (280.9385, 293.1347) -> (281.1313, 293.4236)
  line L1527 (280.8474, 293.0205) -> (280.9385, 293.1347)
  line L1528 (281.2586, 293.6369) -> (281.4025, 293.898)
  line L1529 (281.897, 295.1701) -> (281.8985, 295.3434)
  line L1530 (231.9627, 299.3965) -> (232.2269, 299.6559)
  line L1531 (305.5316, 304.9741) -> (305.8354, 305.2299)
  line L1532 (232.9222, 300.5825) -> (232.9746, 300.7105)
  line L1533 (305.8354, 305.2299) -> (306.1578, 305.5139)
  line L1534 (281.8497, 294.9073) -> (281.8808, 295.0491)
  line L1535 (190.0171, 306.3656) -> (190.2046, 306.0858)
  line L1536 (232.4447, 299.8956) -> (232.6196, 300.1118)
  line L1537 (232.8548, 300.459) -> (232.9222, 300.5825)
  line L1538 (242.0579, 293.386) -> (241.9043, 293.161)
  line L1539 (218.5146, 298.2884) -> (230.3584, 298.2865)
  line L1540 (281.5603, 294.208) -> (281.7289, 294.5685)
  line L1541 (241.764, 292.9293) -> (241.4741, 292.4047)
  line L1542 (242.5919, 294.0076) -> (242.4022, 293.8107)
  line L1543 (281.7289, 294.5685) -> (281.8003, 294.7466)
  line L1544 (232.7551, 300.3009) -> (232.8548, 300.459)
  line L1545 (292.8542, 304.1073) -> (304.1421, 304.1073)
  line L1546 (215.7537, 301.044) -> (216.79, 299.34)
  line L1547 (230.3584, 298.2865) -> (230.5081, 298.3492)
  line L1548 (265.9991, 292.201) -> (279.2627, 292.201)
  line L1549 (230.6547, 298.4238) -> (230.8444, 298.5329)
  line L1550 (281.8537, 295.4187) -> (281.7902, 295.4143)
  line L1551 (232.6927, 301.445) -> (216.3979, 301.4446)
  line L1552 (304.3182, 304.1655) -> (304.5175, 304.2601)
  line L1553 (266.1396, 307.15) -> (265.9991, 292.201)
  line L1554 (241.4042, 292.2612) -> (241.3875, 292.201)
  line L1555 (304.5175, 304.2601) -> (304.7393, 304.3895)
  line L1556 (230.8444, 298.5329) -> (231.0736, 298.6806)
  line L1557 (281.8808, 295.0491) -> (281.897, 295.1701)
  line L1558 (232.6196, 300.1118) -> (232.7551, 300.3009)
  line L1559 (231.6363, 299.1082) -> (231.9627, 299.3965)
  line L1560 (241.4741, 292.4047) -> (241.4042, 292.2612)
  line L1561 (254.6527, 295.3294) -> (254.4599, 295.3391)
  line L1562 (232.9746, 300.7105) -> (232.6927, 301.445)
  line L1563 (281.7902, 295.4143) -> (281.5595, 295.3866)
  line L1564 (280.6917, 295.3175) -> (269.1924, 295.376)
  line L1565 (242.7924, 294.1926) -> (242.5919, 294.0076)
  line L1566 (216.79, 299.34) -> (218.5146, 298.2884)
  line L1567 (254.8555, 295.3497) -> (254.8011, 295.3348)
  line L1568 (216.3979, 301.4446) -> (215.7537, 301.044)
  line L1569 (242.4022, 293.8107) -> (242.224, 293.603)
  line L1570 (281.4025, 293.898) -> (281.5603, 294.208)
  line L1571 (269.05, 307.1326) -> (266.1396, 307.15)
  line L1572 (242.224, 293.603) -> (242.0579, 293.386)
  line L1573 (290.349, 301.4319) -> (290.349, 292.201)
  line L1574 (305.2471, 304.7479) -> (305.5316, 304.9741)
  line L1575 (269.1924, 295.376) -> (269.05, 307.1326)
  line L1576 (281.1313, 293.4236) -> (281.2586, 293.6369)
  line L1577 (231.0736, 298.6806) -> (231.3388, 298.8709)
  line L1578 (231.3388, 298.8709) -> (231.6363, 299.1082)
  line L1579 (281.8003, 294.7466) -> (281.8497, 294.9073)
  line L1580 (208.3451, 275.8168) -> (210.3054, 276.2177)
  line L1581 (306.1578, 305.5139) -> (306.4597, 305.7743)
  line L1582 (231.8829, 305.1424) -> (232.078, 305.3312)
  line L1583 (231.0361, 304.4748) -> (231.2882, 304.6523)
  line L1584 (231.5715, 304.8735) -> (231.8829, 305.1424)
  line L1585 (291.0104, 305.0871) -> (292.8542, 304.1073)
  line L1586 (223.9511, 278.3387) -> (225.8775, 278.5435)
  line L1587 (232.8454, 306.557) -> (232.888, 306.6999)
  line L1588 (227.8058, 278.7321) -> (229.7354, 278.9081)
  line L1589 (222.0273, 278.1136) -> (223.9511, 278.3387)
  line L1590 (232.9186, 306.8301) -> (232.9495, 307.0464)
  line L1591 (232.5229, 305.8895) -> (232.6294, 306.0677)
  line L1592 (205.4163, 275.1637) -> (206.3909, 275.3886)
  line L1593 (216.2142, 277.276) -> (218.1901, 277.5872)
  line L1594 (198.2889, 273.2034) -> (198.3595, 273.2155)
  line L1595 (202.5045, 274.4426) -> (203.473, 274.6909)
  line L1596 (203.473, 274.6909) -> (204.4437, 274.9312)
  line L1597 (230.4999, 304.1659) -> (230.6387, 304.2355)
  line L1598 (204.4437, 274.9312) -> (205.4163, 275.1637)
  line L1599 (306.7152, 305.9894) -> (306.8202, 306.0834)
  line L1600 (307.0177, 306.3278) -> (307.0177, 307.2464)
  line L1601 (198.59, 273.2787) -> (199.41, 273.5402)
  line L1602 (230.8186, 304.3372) -> (231.0361, 304.4748)
  line L1603 (200.0008, 273.727) -> (200.713, 273.9435)
  line L1604 (232.078, 305.3312) -> (232.2487, 305.5197)
  line L1605 (306.4597, 305.7743) -> (306.7152, 305.9894)
  line L1606 (232.2487, 305.5197) -> (232.3965, 305.7063)
  line L1607 (307.0177, 307.2464) -> (290.1046, 307.2644)
  line L1608 (200.713, 273.9435) -> (201.5474, 274.184)
  line L1609 (220.1068, 277.8644) -> (222.0273, 278.1136)
  line L1610 (306.8202, 306.0834) -> (306.907, 306.1702)
  line L1611 (212.271, 276.5932) -> (214.2409, 276.9454)
  line L1612 (218.1901, 277.5872) -> (220.1068, 277.8644)
  line L1613 (306.9736, 306.2512) -> (307.0177, 306.3278)
  line L1614 (232.9495, 307.0464) -> (232.9507, 307.1936)
  line L1615 (216.0181, 307.2593) -> (215.7639, 306.848)
  line L1616 (230.3584, 304.1073) -> (230.4999, 304.1659)
  line L1617 (289.8287, 306.8181) -> (291.0104, 305.0871)
  line L1618 (232.888, 306.6999) -> (232.9186, 306.8301)
  line L1619 (201.5474, 274.184) -> (202.5045, 274.4426)
  line L1620 (210.3054, 276.2177) -> (212.271, 276.5932)
  line L1621 (225.8775, 278.5435) -> (227.8058, 278.7321)
  line L1622 (232.9344, 307.2593) -> (216.0181, 307.2593)
  line L1623 (230.6387, 304.2355) -> (230.8186, 304.3372)
  line L1624 (199.41, 273.5402) -> (200.0008, 273.727)
  line L1625 (215.7639, 306.848) -> (216.79, 305.1608)
  line L1626 (304.9827, 304.5526) -> (305.2471, 304.7479)
  line L1627 (232.3965, 305.7063) -> (232.5229, 305.8895)
  line L1628 (198.3595, 273.2155) -> (198.59, 273.2787)
  line L1629 (229.7354, 278.9081) -> (233.5958, 279.2384)
  line L1630 (214.2409, 276.9454) -> (216.2142, 277.276)
  line L1631 (232.9439, 307.2374) -> (232.9344, 307.2593)
  line L1632 (206.3909, 275.3886) -> (208.3451, 275.8168)
  line L1633 (198.2479, 273.2051) -> (198.2889, 273.2034)
  line L1634 (232.7891, 306.403) -> (232.8454, 306.557)
  line L1635 (231.2882, 304.6523) -> (231.5715, 304.8735)
  line L1636 (218.5146, 304.1093) -> (230.3584, 304.1073)
  line L1637 (306.907, 306.1702) -> (306.9736, 306.2512)
  line L1638 (232.6294, 306.0677) -> (232.7176, 306.2394)
  line L1639 (290.1046, 307.2644) -> (289.8287, 306.8181)
  line L1640 (232.7176, 306.2394) -> (232.7891, 306.403)
  line L1641 (269.0626, 278.9314) -> (270.9714, 278.7417)
  line L1642 (235.0904, 279.3888) -> (235.8378, 279.4607)
  line L1643 (278.4723, 277.8431) -> (279.8257, 277.6455)
  line L1644 (303.3837, 277.3796) -> (303.395, 277.4088)
  line L1645 (287.9091, 276.228) -> (289.2489, 275.9534)
  line L1646 (303.3474, 277.3231) -> (303.3837, 277.3796)
  line L1647 (300.0051, 273.2104) -> (300.0819, 273.1791)
  line L1648 (300.5641, 273.6636) -> (300.8452, 274.0242)
  line L1649 (303.141, 277.695) -> (303.0392, 277.7704)
  line L1650 (283.876, 276.9863) -> (285.2225, 276.7445)
  line L1651 (297.1561, 274.1437) -> (297.6681, 274.0132)
  line L1652 (274.4044, 278.3694) -> (275.7616, 278.2051)
  line L1653 (303.0392, 277.7704) -> (302.9167, 277.8478)
  line L1654 (289.2489, 275.9534) -> (290.5863, 275.6679)
  line L1655 (302.5493, 277.9917) -> (302.1683, 278.1223)
  line L1656 (299.0098, 273.6131) -> (299.2928, 273.51)
  line L1657 (302.1683, 278.1223) -> (301.6549, 278.2891)
  line L1658 (301.6549, 278.2891) -> (301.0089, 278.4898)
  line L1659 (294.5823, 274.7461) -> (295.6116, 274.5048)
  line L1660 (270.9714, 278.7417) -> (273.0463, 278.5226)
  line L1661 (300.8452, 274.0242) -> (301.6101, 275.03)
  line L1662 (302.9167, 277.8478) -> (302.7987, 277.8995)
  line L1663 (273.0463, 278.5226) -> (274.4044, 278.3694)
  line L1664 (263.0936, 279.4207) -> (264.3354, 279.3361)
  line L1665 (297.6681, 274.0132) -> (298.1774, 273.8733)
  line L1666 (282.5277, 277.217) -> (283.876, 276.9863)
  line L1667 (298.6833, 273.7214) -> (299.0098, 273.6131)
  line L1668 (285.2225, 276.7445) -> (286.5669, 276.4917)
  line L1669 (264.3354, 279.3361) -> (265.7443, 279.2273)
  line L1670 (300.0819, 273.1791) -> (300.1197, 273.1713)
  line L1671 (216.79, 305.1608) -> (218.5146, 304.1093)
  line L1672 (300.1197, 273.1713) -> (300.1526, 273.1907)
  line L1673 (279.8257, 277.6455) -> (281.1775, 277.4368)
  line L1674 (290.5863, 275.6679) -> (291.9211, 275.3715)
  line L1675 (303.2883, 277.5588) -> (303.2236, 277.6237)
  line L1676 (303.2029, 277.1278) -> (303.3474, 277.3231)
  line L1677 (296.6422, 274.2674) -> (297.1561, 274.1437)
  line L1678 (293.2531, 275.0642) -> (294.5823, 274.7461)
  line L1679 (286.5669, 276.4917) -> (287.9091, 276.228)
  line L1680 (236.212, 279.4893) -> (236.5867, 279.5107)
  line L1681 (300.1526, 273.1907) -> (300.2019, 273.2355)
  line L1682 (295.6116, 274.5048) -> (296.6422, 274.2674)
  line L1683 (299.7314, 273.3315) -> (300.0051, 273.2104)
  line L1684 (262.0192, 279.4822) -> (263.0936, 279.4207)
  line L1685 (298.1774, 273.8733) -> (298.6833, 273.7214)
  line L1686 (299.2928, 273.51) -> (299.7314, 273.3315)
  line L1687 (267.3201, 279.0928) -> (269.0626, 278.9314)
  line L1688 (303.3693, 277.4574) -> (303.2883, 277.5588)
  line L1689 (303.2236, 277.6237) -> (303.141, 277.695)
  line L1690 (234.3434, 279.3098) -> (235.0904, 279.3888)
  line L1691 (275.7616, 278.2051) -> (277.1176, 278.0297)
  line L1692 (301.6101, 275.03) -> (302.6491, 276.4044)
  line L1693 (232.9507, 307.1936) -> (232.9439, 307.2374)
  line L1694 (281.1775, 277.4368) -> (282.5277, 277.217)
  line L1695 (300.2019, 273.2355) -> (300.3499, 273.4002)
  line L1696 (277.1176, 278.0297) -> (278.4723, 277.8431)
  line L1697 (302.6491, 276.4044) -> (303.2029, 277.1278)
  line L1698 (303.395, 277.4088) -> (303.3693, 277.4574)
  line L1699 (302.7987, 277.8995) -> (302.5493, 277.9917)
  line L1700 (291.9211, 275.3715) -> (293.2531, 275.0642)
  line L1701 (300.3499, 273.4002) -> (300.5641, 273.6636)
  line L1702 (233.5958, 279.2384) -> (234.3434, 279.3098)
  line L1703 (236.5867, 279.5107) -> (261.1125, 279.5221)
  line L1704 (235.8378, 279.4607) -> (236.212, 279.4893)
  line L1705 (294.3197, 280.238) -> (293.1141, 280.4977)
  line L1706 (216.7961, 282.3936) -> (215.645, 282.2408)
  line L1707 (198.1417, 278.6743) -> (196.2186, 278.1024)
  line L1708 (195.1112, 277.5316) -> (195.1011, 277.4923)
  line L1709 (295.4381, 279.9839) -> (294.3197, 280.238)
  line L1710 (219.1849, 282.6854) -> (217.9761, 282.542)
  line L1711 (199.2589, 278.9946) -> (198.1417, 278.6743)
  line L1712 (228.4526, 283.5204) -> (227.0424, 283.4219)
  line L1713 (280.3205, 282.5523) -> (278.3271, 282.7786)
  line L1714 (296.4692, 279.7372) -> (295.4381, 279.9839)
  line L1715 (234.5106, 283.9417) -> (233.5373, 283.8609)
  line L1716 (301.0089, 278.4898) -> (300.2296, 278.7222)
  line L1717 (210.3217, 281.4227) -> (208.3944, 281.0774)
  line L1718 (225.6609, 283.3159) -> (224.3081, 283.2026)
  line L1719 (220.4225, 282.8236) -> (219.1849, 282.6854)
  line L1720 (293.1141, 280.4977) -> (291.8211, 280.761)
  line L1721 (271.0467, 283.4676) -> (269.5312, 283.602)
  line L1722 (224.3081, 283.2026) -> (222.9841, 283.0826)
  line L1723 (288.9728, 281.2913) -> (287.4175, 281.5546)
  line L1724 (231.9979, 283.7465) -> (229.8917, 283.6109)
  line L1725 (265.7443, 279.2273) -> (267.3201, 279.0928)
  line L1726 (217.9761, 282.542) -> (216.7961, 282.3936)
  line L1727 (278.3271, 282.7786) -> (276.246, 282.992)
  line L1728 (252.9104, 284.3296) -> (234.9187, 283.9767)
  line L1729 (268.0144, 283.7196) -> (252.9104, 284.3296)
  line L1730 (200.4921, 279.3277) -> (199.2589, 278.9946)
  line L1731 (300.2296, 278.7222) -> (299.3168, 278.9841)
  line L1732 (261.1125, 279.5221) -> (262.0192, 279.4822)
  line L1733 (227.0424, 283.4219) -> (225.6609, 283.3159)
  line L1734 (214.5226, 282.0839) -> (212.3645, 281.7592)
  line L1735 (204.8864, 280.373) -> (203.3059, 280.0199)
  line L1736 (233.5373, 283.8609) -> (231.9979, 283.7465)
  line L1737 (201.8411, 279.6705) -> (200.4921, 279.3277)
  line L1738 (298.2698, 279.2731) -> (297.4131, 279.4996)
  line L1739 (215.645, 282.2408) -> (214.5226, 282.0839)
  line L1740 (195.4958, 277.8677) -> (195.3395, 277.767)
  line L1741 (285.7746, 281.8142) -> (284.0442, 282.0682)
  line L1742 (196.2186, 278.1024) -> (195.7066, 277.9435)
  line L1743 (290.4407, 281.0262) -> (288.9728, 281.2913)
  line L1744 (269.5312, 283.602) -> (268.0144, 283.7196)
  line L1745 (287.4175, 281.5546) -> (285.7746, 281.8142)
  line L1746 (234.9187, 283.9767) -> (234.5106, 283.9417)
  line L1747 (195.7066, 277.9435) -> (195.4958, 277.8677)
  line L1748 (203.3059, 280.0199) -> (201.8411, 279.6705)